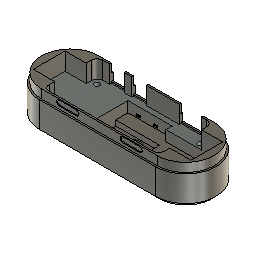
OP_Lower (Autodesk Fusion 360 design; units mm, degrees)
Autodesk Fusion 360 part; units mm, degrees
sketch "Sketch1" plane through (0, 0, 0) normal (0, 0, 1) x (1, 0, 0)
  line L0 (32.75, -17.25) -> (-32.75, -17.25)
  line L1 (-32.75, 17.25) -> (32.75, 17.25)
  arc A0 (-32.75, 17.25) -> (-32.75, -17.25) centre (-32.75, 0) ccw
  arc A1 (32.75, -17.25) -> (32.75, 17.25) centre (32.75, 0) ccw
extrude "Extrude1" add sketch "Sketch1" along normal blind 18
sketch "Sketch2" plane through (0, 0, 18) normal (0, 0, 1) x (-1, 0, 0)
  arc A0 (32.75, -17.25) -> (32.75, 17.25) centre (32.75, 0) ccw
  line L0 (32.75, 17.25) -> (-32.75, 17.25)
  arc A1 (-32.75, 17.25) -> (-32.75, -17.25) centre (-32.75, 0) ccw
  line L1 (-32.75, -17.25) -> (32.75, -17.25)
  line L2 (-12.5, -12.5) -> (12.5, -12.5)
  line L3 (12.5, -12.5) -> (12.5, 12.5)
  line L4 (12.5, 12.5) -> (-12.5, 12.5)
  line L5 (-12.5, 12.5) -> (-12.5, -12.5)
  line L6 (-12.5, -12.5) -> (12.5, 12.5) construction
  line L7 (12.5, -12.5) -> (-12.5, 12.5) construction
  dimension "d9" = 25
  dimension "d10" = 25
  constraint horizontal L2
  constraint perpendicular L2 L3
  constraint parallel L2 L4
  constraint parallel L3 L5
  constraint coincident L6 origin
  constraint coincident L7 origin
  measures "d9" distance of L3.end L4.end
  measures "d10" distance of L2.end L3.end
extrude "Extrude2" cut sketch "Sketch2" against normal blind 15 contours L2 L3 L4 L5
sketch "Sketch3" plane through (0, 0, 3) normal (0, 0, 1) x (-1, 0, 0)
  line L0 (-12.5, 12.5) -> (-12.5, -12.5)
  line L1 (-12.5, -12.5) -> (12.5, -12.5)
  line L2 (12.5, -12.5) -> (12.5, 12.5)
  line L3 (12.5, 12.5) -> (-12.5, 12.5)
sketch "Sketch4" plane through (0, 0, 3) normal (0, 0, 1) x (-1, 0, 0)
  line L0 (-12.5, 12.5) -> (-12.5, -12.5)
  line L1 (-12.5, -12.5) -> (12.5, -12.5)
  line L2 (12.5, -12.5) -> (12.5, 12.5)
  line L3 (12.5, 12.5) -> (-12.5, 12.5)
  line L4 (12.5, 0) -> (12.5, -5.5) construction
  line L5 (12.5, -5.5) -> (-12.5, -5.5)
  line L6 (12.5, 0) -> (12.5, 5.5) construction
  line L7 (12.5, 5.5) -> (-12.5, 5.5)
  constraint midpoint L2 L4.start
  constraint parallel L2 L4
  constraint coincident L0 L5.end
  constraint perpendicular L0 L5
  constraint perpendicular L5 L6
  constraint coincident L0 L7.end
  constraint perpendicular L0 L7
extrude "Extrude4" add sketch "Sketch4" along normal blind 3 contours L0 L2 L3 L7 | L0 L1 L2 L5
sketch "Sketch5" plane through (0, 0, 18) normal (0, 0, 1) x (-1, 0, 0)
  line L0 (12.5, -12.5) -> (-12.5, -12.5)
  line L1 (-12.5, -12.5) -> (-12.5, 12.5)
  line L2 (-12.5, 12.5) -> (12.5, 12.5)
  line L3 (12.5, 12.5) -> (12.5, -12.5)
  arc A0 (32.75, -17.25) -> (32.75, 17.25) centre (32.75, 0) ccw
  line L4 (32.75, 17.25) -> (-32.75, 17.25)
  arc A1 (-32.75, 17.25) -> (-32.75, -17.25) centre (-32.75, 0) ccw
  line L5 (-32.75, -17.25) -> (32.75, -17.25)
  line L6 (29.5, -15.25) -> (25.75, -15.25)
  arc A2 (29.5, -15.25) -> (32.75, -12) centre (29.5, -12) ccw
  line L7 (32.75, 12) -> (32.75, -12)
  arc A3 (32.75, 12) -> (29.5, 15.25) centre (29.5, 12) ccw
  line L8 (-29.5, 15.25) -> (29.5, 15.25)
  arc A4 (-29.5, 15.25) -> (-32.75, 12) centre (-29.5, 12) ccw
  line L9 (-32.75, -12) -> (-32.75, 12)
  arc A5 (-32.75, -12) -> (-29.5, -15.25) centre (-29.5, -12) ccw
  line L10 (-26.35, -15.25) -> (-29.5, -15.25)
  line L11 (-13.85, -17.25) -> (-26.35, -17.25)
  line L12 (-26.35, -17.25) -> (-26.35, -15.25)
  line L13 (-13.85, -15.25) -> (-13.85, -17.25)
  line L14 (4.65, -15.25) -> (-13.85, -15.25)
  line L15 (4.65, -18.25) -> (4.65, -15.25)
  line L16 (13.15, -18.25) -> (4.65, -18.25)
  line L17 (13.15, -15.25) -> (13.15, -18.25)
  line L18 (17.25, -15.25) -> (13.15, -15.25)
  line L19 (17.25, -18.25) -> (17.25, -15.25)
  line L20 (25.75, -18.25) -> (17.25, -18.25)
  line L21 (25.75, -15.25) -> (25.75, -18.25)
  line L22 (32.75, 0) -> (32.75, -9) construction
  line L23 (32.75, 0) -> (32.75, 9) construction
  line L24 (32.75, -9) -> (44.75, -9)
  line L25 (32.75, 9) -> (44.75, 9)
  line L26 (44.75, -9) -> (44.75, 9)
  line L27 (-32.75, 0) -> (-32.75, -9) construction
  line L28 (-32.75, 0) -> (-32.75, 9) construction
  line L29 (-32.75, -9) -> (-44.75, -9)
  line L30 (-32.75, 9) -> (-44.75, 9)
  line L31 (-44.75, 9) -> (-44.75, -9)
  dimension "d20" = 9
  dimension "d21" = 9
  dimension "d23" = 12
  dimension "d26" = 12
  constraint coincident A0.centre L22.start
  constraint parallel L7 L22
  constraint parallel L7 L23
  constraint perpendicular L22 L24
  constraint perpendicular L7 L25
  constraint perpendicular L25 L26
  constraint coincident A1.centre L27.start
  constraint perpendicular L25 L27
  constraint parallel L9 L28
  constraint perpendicular L9 L29
  constraint perpendicular L9 L30
  constraint perpendicular L29 L31
  measures "d20" distance of A0.centre L22.end
  measures "d21" distance of A0.centre L23.end
  measures "d23" distance of L23.end L25.end
  measures "d26" distance of L27.end L29.end
extrude "Extrude5" cut sketch "Sketch5" against normal blind 5 contours L5 L6 A2 L7 A3 L8 A4 L9 A5 L10 L11 L12 L13 L14 L15 L17 L18 L19 L21 | L7 L24 L25 L26 | L9 L29 L30 L31
sketch "Sketch6" plane through (0, 0, 6) normal (0, 0, 1) x (-1, 0, 0)
  line L0 (12.5, 12.5) -> (-12.5, 12.5)
  line L1 (-12.5, 12.5) -> (-12.5, 5.5)
  line L2 (-12.5, 5.5) -> (12.5, 5.5)
  line L3 (12.5, 5.5) -> (12.5, 12.5)
  line L4 (12.5, 5.5) -> (6.5, 5.5) construction
  line L5 (6.5, 5.5) -> (6.5, 12.5)
  dimension "d30" = 6
  constraint coincident L2.end L3.start
  constraint perpendicular L3 L4
  constraint coincident L0 L5.end
  constraint perpendicular L0 L5
  measures "d30" distance of L2.end L4.end
extrude "Extrude6" cut sketch "Sketch6" against normal blind 1.5 contours L0 L2 L3 L5
sketch "Sketch7" plane through (0, 0, 13) normal (0, 0, 1) x (-1, 0, 0)
  line L0 (-12.5, 12.5) -> (12.5, 12.5)
  line L1 (12.5, 12.5) -> (12.5, -12.5)
  line L2 (12.5, -12.5) -> (-12.5, -12.5)
  line L3 (-12.5, -12.5) -> (-12.5, 12.5)
  line L4 (-32.75, 9) -> (-44.75, 9)
  line L5 (-44.75, 9) -> (-44.75, -9)
  line L6 (-44.75, -9) -> (-32.75, -9)
  line L7 (-32.75, -9) -> (-32.75, -12)
  arc A0 (-32.75, -12) -> (-29.5, -15.25) centre (-29.5, -12) ccw
  line L8 (-29.5, -15.25) -> (-26.35, -15.25)
  line L9 (-26.35, -15.25) -> (-26.35, -17.25)
  line L10 (-26.35, -17.25) -> (-13.85, -17.25)
  line L11 (-13.85, -17.25) -> (-13.85, -15.25)
  line L12 (-13.85, -15.25) -> (4.65, -15.25)
  line L13 (4.65, -15.25) -> (4.65, -17.25)
  line L14 (4.65, -17.25) -> (13.15, -17.25)
  line L15 (13.15, -17.25) -> (13.15, -15.25)
  line L16 (13.15, -15.25) -> (17.25, -15.25)
  line L17 (17.25, -15.25) -> (17.25, -17.25)
  line L18 (17.25, -17.25) -> (25.75, -17.25)
  line L19 (25.75, -17.25) -> (25.75, -15.25)
  line L20 (25.75, -15.25) -> (29.5, -15.25)
  arc A1 (29.5, -15.25) -> (32.75, -12) centre (29.5, -12) ccw
  line L21 (32.75, -12) -> (32.75, -9)
  line L22 (32.75, -9) -> (44.75, -9)
  line L23 (44.75, -9) -> (44.75, 9)
  line L24 (44.75, 9) -> (32.75, 9)
  line L25 (32.75, 9) -> (32.75, 12)
  arc A2 (32.75, 12) -> (29.5, 15.25) centre (29.5, 12) ccw
  line L26 (29.5, 15.25) -> (-29.5, 15.25)
  arc A3 (-29.5, 15.25) -> (-32.75, 12) centre (-29.5, 12) ccw
  line L27 (-32.75, 12) -> (-32.75, 9)
  line L28 (0, 15.25) -> (26.5, 15.25) construction
  line L29 (0, 15.25) -> (-26.5, 15.25) construction
  line L30 (26.5, 15.25) -> (26.5, 9.25)
  line L31 (-26.5, 15.25) -> (-26.5, 9.25)
  line L32 (26.5, 9.25) -> (-26.5, 9.25)
  dimension "d33" = 26.5
  dimension "d34" = 26.5
  dimension "d35" = 6
  dimension "d36" = 6
  constraint midpoint L26 L28.start
  constraint parallel L26 L28
  constraint parallel L26 L29
  constraint perpendicular L28 L30
  constraint perpendicular L29 L31
  measures "d33" distance of L28.start L28.end
  measures "d34" distance of L28.start L29.end
  measures "d35" distance of L28.end L30.end
  measures "d36" distance of L29.end L31.end
extrude "Extrude7" cut sketch "Sketch7" against normal blind 4 contours L0 L1 L3 L26 L30 L31 L32
sketch "Sketch8" plane through (0, 0, 13) normal (0, 0, 1) x (-1, 0, 0)
  line L0 (26.5, 9.25) -> (12.5, 9.25)
  line L1 (12.5, 9.25) -> (12.5, -12.5)
  line L2 (12.5, -12.5) -> (-12.5, -12.5)
  line L3 (-12.5, -12.5) -> (-12.5, 9.25)
  line L4 (-12.5, 9.25) -> (-26.5, 9.25)
  line L5 (-26.5, 9.25) -> (-26.5, 15.25)
  line L6 (-26.5, 15.25) -> (-29.5, 15.25)
  arc A0 (-29.5, 15.25) -> (-32.75, 12) centre (-29.5, 12) ccw
  line L7 (-32.75, 12) -> (-32.75, 9)
  line L8 (-32.75, 9) -> (-44.75, 9)
  line L9 (-44.75, 9) -> (-44.75, -9)
  line L10 (-44.75, -9) -> (-32.75, -9)
  line L11 (-32.75, -9) -> (-32.75, -12)
  arc A1 (-32.75, -12) -> (-29.5, -15.25) centre (-29.5, -12) ccw
  line L12 (-29.5, -15.25) -> (-26.35, -15.25)
  line L13 (-26.35, -15.25) -> (-26.35, -17.25)
  line L14 (-26.35, -17.25) -> (-13.85, -17.25)
  line L15 (-13.85, -17.25) -> (-13.85, -15.25)
  line L16 (-13.85, -15.25) -> (4.65, -15.25)
  line L17 (4.65, -15.25) -> (4.65, -17.25)
  line L18 (4.65, -17.25) -> (13.15, -17.25)
  line L19 (13.15, -17.25) -> (13.15, -15.25)
  line L20 (13.15, -15.25) -> (17.25, -15.25)
  line L21 (17.25, -15.25) -> (17.25, -17.25)
  line L22 (17.25, -17.25) -> (25.75, -17.25)
  line L23 (25.75, -17.25) -> (25.75, -15.25)
  line L24 (25.75, -15.25) -> (29.5, -15.25)
  arc A2 (29.5, -15.25) -> (32.75, -12) centre (29.5, -12) ccw
  line L25 (32.75, -12) -> (32.75, -9)
  line L26 (32.75, -9) -> (44.75, -9)
  line L27 (44.75, -9) -> (44.75, 9)
  line L28 (44.75, 9) -> (32.75, 9)
  line L29 (32.75, 9) -> (32.75, 12)
  arc A3 (32.75, 12) -> (29.5, 15.25) centre (29.5, 12) ccw
  line L30 (29.5, 15.25) -> (26.5, 15.25)
  line L31 (26.5, 15.25) -> (26.5, 9.25)
  line L32 (-32.75, -9) -> (-12.5, -9)
  line L33 (-32.75, 9) -> (-12.5, 9)
  constraint horizontal L32
  constraint coincident L10.end L11.start
  constraint coincident L3 L32.end
  constraint horizontal L33
  constraint coincident L7.end L8.start
  constraint coincident L3 L33.end
extrude "Extrude8" cut sketch "Sketch8" against normal up to surface (7 mm away) contours L3 L8 L9 L10 L32 L33
sketch "Sketch9" plane through (0, 0, 13) normal (0, 0, 1) x (-1, 0, 0)
  line L0 (-32.75, 9) -> (-12.5, 9)
  line L1 (-12.5, 9) -> (-12.5, 9.25)
  line L2 (-12.5, 9.25) -> (-26.5, 9.25)
  line L3 (-26.5, 9.25) -> (-26.5, 15.25)
  line L4 (-26.5, 15.25) -> (-29.5, 15.25)
  arc A0 (-29.5, 15.25) -> (-32.75, 12) centre (-29.5, 12) ccw
  line L5 (-32.75, 12) -> (-32.75, 9)
  line L6 (-26.5, 9.25) -> (-26.5, 9)
  constraint vertical L6
  constraint coincident L2.end L3.start
  constraint coincident L0 L6.end
extrude "Extrude9" cut sketch "Sketch9" against normal up to surface (7 mm away) contours L0 L1 L2 L6
sketch "Sketch10" plane through (0, 12.5, 0) normal (0, -1, 0) x (1, 0, 0)
  line L0 (12.5, 13) -> (-12.5, 13)
  line L1 (-12.5, 13) -> (-12.5, 6)
  line L2 (-12.5, 6) -> (12.5, 6)
  line L3 (12.5, 6) -> (12.5, 13)
  line L4 (-12.5, 6) -> (-7.5, 6) construction
  line L5 (-7.5, 6) -> (-7.5, 7) construction
  line L6 (-7.5, 7) -> (-5.5, 7)
  line L7 (-5.5, 7) -> (-5.5, 8)
  line L8 (-5.5, 8) -> (-7.5, 8)
  line L9 (-7.5, 8) -> (-7.5, 7)
  line L10 (-5.5, 7) -> (2.5, 7) construction
  line L11 (2.5, 7) -> (4.5, 7)
  line L12 (4.5, 7) -> (4.5, 8)
  line L13 (4.5, 8) -> (2.5, 8)
  line L14 (2.5, 8) -> (2.5, 7)
  dimension "d44" = 1
  dimension "d45" = 2
  dimension "d46" = 1
  dimension "d47" = 8
  dimension "d48" = 2
  dimension "d49" = 1
  constraint coincident L1.end L2.start
  constraint perpendicular L1 L4
  constraint perpendicular L4 L5
  constraint horizontal L6
  constraint vertical L7
  constraint horizontal L8
  constraint vertical L9
  constraint perpendicular L7 L10
  constraint horizontal L11
  constraint vertical L12
  constraint horizontal L13
  constraint vertical L14
  measures "d44" distance of L4.end L5.end
  measures "d45" distance of L5.end L6.end
  measures "d46" distance of L5.end L8.end
  measures "d47" distance of L6.end L10.end
  measures "d48" distance of L10.end L11.end
  measures "d49" distance of L10.end L13.end
extrude "Extrude10" add sketch "Sketch10" along normal blind 0.5 contours L6 L7 L8 L9 | L11 L12 L13 L14
chamfer "Chamfer1" distance 0.2 distance2 0.2 4 edges at (-6.5, 12, 8) (-6.5, 12, 7) (3.5, 12, 8) (3.5, 12, 7) measured on face at (-6.8333, 12, 7.6667) measured on face at (-6.8333, 12, 7.6667) measured on face at (3.1667, 12, 7.6667) measured on face at (3.1667, 12, 7.6667)
sketch "Sketch11" plane through (0, -12.5, 0) normal (0, 1, 0) x (-1, 0, 0)
  line L0 (12.5, 9) -> (-12.5, 9)
  line L1 (-12.5, 9) -> (-12.5, 6)
  line L2 (-12.5, 6) -> (6.5, 6)
  line L3 (6.5, 6) -> (6.5, 4.5)
  line L4 (6.5, 4.5) -> (12.5, 4.5)
  line L5 (12.5, 4.5) -> (12.5, 9)
  line L6 (6.5, 6) -> (12.5, 6) construction
  line L7 (12.5, 6) -> (12.5, 7) construction
  line L8 (12.5, 7) -> (7.5, 7) construction
  line L9 (7.5, 7) -> (5.5, 7)
  line L10 (5.5, 7) -> (5.5, 8)
  line L11 (5.5, 8) -> (7.5, 8)
  line L12 (7.5, 8) -> (7.5, 7)
  line L13 (5.5, 7) -> (-2.5, 7) construction
  line L14 (-2.5, 7) -> (-4.5, 7)
  line L15 (-4.5, 7) -> (-4.5, 8)
  line L16 (-4.5, 8) -> (-2.5, 8)
  line L17 (-2.5, 8) -> (-2.5, 7)
  dimension "d54" = 1
  dimension "d55" = 5
  dimension "d56" = 2
  dimension "d57" = 1
  dimension "d58" = 8
  dimension "d59" = 2
  dimension "d60" = 1
  constraint coincident L2.end L3.start
  constraint coincident L5 L6.end
  constraint perpendicular L5 L6
  constraint perpendicular L6 L7
  constraint perpendicular L7 L8
  constraint horizontal L9
  constraint vertical L10
  constraint horizontal L11
  constraint vertical L12
  constraint perpendicular L10 L13
  constraint horizontal L14
  constraint vertical L15
  constraint horizontal L16
  constraint vertical L17
  measures "d54" distance of L6.end L7.end
  measures "d55" distance of L7.end L8.end
  measures "d56" distance of L8.end L9.end
  measures "d57" distance of L8.end L11.end
  measures "d58" distance of L9.end L13.end
  measures "d59" distance of L13.end L14.end
  measures "d60" distance of L13.end L16.end
extrude "Extrude11" add sketch "Sketch11" along normal blind 0.5 contours L9 L10 L11 L12 | L14 L15 L16 L17
chamfer "Chamfer2" distance 0.2 distance2 0.2 4 edges at (-6.5, -12, 8) (-6.5, -12, 7) (3.5, -12, 8) (3.5, -12, 7) measured on face at (-6.1667, -12, 7.6667) measured on face at (-6.1667, -12, 7.6667) measured on face at (3.8333, -12, 7.6667) measured on face at (3.8333, -12, 7.6667)
sketch "Sketch13" plane through (0, 0, 18) normal (0, 0, 1) x (-1, 0, 0)
  line L0 (-26.35, -17.25) -> (-26.35, -15.25)
  line L1 (-26.35, -15.25) -> (-29.5, -15.25)
  arc A0 (-32.75, -12) -> (-29.5, -15.25) centre (-29.5, -12) ccw
  line L2 (-32.75, -12) -> (-32.75, -9)
  line L3 (-32.75, -9) -> (-44.75, -9)
  line L4 (-44.75, -9) -> (-44.75, 9)
  line L5 (-44.75, 9) -> (-32.75, 9)
  line L6 (-32.75, 9) -> (-32.75, 12)
  arc A1 (-29.5, 15.25) -> (-32.75, 12) centre (-29.5, 12) ccw
  line L7 (-29.5, 15.25) -> (29.5, 15.25)
  arc A2 (32.75, 12) -> (29.5, 15.25) centre (29.5, 12) ccw
  line L8 (32.75, 12) -> (32.75, 9)
  line L9 (32.75, 9) -> (44.75, 9)
  line L10 (44.75, 9) -> (44.75, -9)
  line L11 (44.75, -9) -> (32.75, -9)
  line L12 (32.75, -9) -> (32.75, -12)
  arc A3 (29.5, -15.25) -> (32.75, -12) centre (29.5, -12) ccw
  line L13 (29.5, -15.25) -> (25.75, -15.25)
  line L14 (25.75, -15.25) -> (25.75, -17.25)
  line L15 (25.75, -17.25) -> (32.75, -17.25)
  arc A4 (32.75, -17.25) -> (32.75, 17.25) centre (32.75, 0) ccw
  line L16 (32.75, 17.25) -> (-32.75, 17.25)
  arc A5 (-32.75, 17.25) -> (-32.75, -17.25) centre (-32.75, 0) ccw
  line L17 (-32.75, -17.25) -> (-26.35, -17.25)
  line L18 (25.75, -16.25) -> (32.75, -16.25)
  arc A6 (32.75, -16.25) -> (32.75, 16.25) centre (32.75, 0) ccw
  line L19 (32.75, 16.25) -> (-32.75, 16.25)
  arc A7 (-32.75, 16.25) -> (-32.75, -16.25) centre (-32.75, 0) ccw
  line L20 (-32.75, -16.25) -> (-26.35, -16.25)
  line L21 (25.75, -15.25) -> (32.75, -15.25)
  arc A8 (32.75, -15.25) -> (32.75, 15.25) centre (32.75, 0) ccw
  line L22 (32.75, 15.25) -> (-32.75, 15.25)
  arc A9 (-32.75, 15.25) -> (-32.75, -15.25) centre (-32.75, 0) ccw
  line L23 (-32.75, -15.25) -> (-26.35, -15.25)
  dimension "d79" = -1
  dimension "d80" = -2
extrude "Extrude13" add sketch "Sketch13" along normal blind 2 contours L0 L1 L7 L13 L14 L18 A6 L19 A7 L20 L21 A8 L22 A9 L23
sketch "Sketch14" plane through (0, 0, 18) normal (0, 0, 1) x (-1, 0, 0)
  line L0 (-13.85, -15.25) -> (-13.85, -17.25)
  line L1 (-13.85, -17.25) -> (4.65, -17.25)
  line L2 (4.65, -17.25) -> (4.65, -15.25)
  line L3 (4.65, -15.25) -> (-13.85, -15.25)
  line L4 (4.65, -16.25) -> (-13.85, -16.25)
  constraint midpoint L2 L4.start
  constraint midpoint L0 L4.end
extrude "Extrude14" add sketch "Sketch14" along normal blind 2 contours L0 L2 L3 L4
sketch "Sketch15" plane through (0, 0, 18) normal (0, 0, 1) x (-1, 0, 0)
  line L0 (13.15, -15.25) -> (13.15, -17.25)
  line L1 (13.15, -17.25) -> (17.25, -17.25)
  line L2 (17.25, -17.25) -> (17.25, -15.25)
  line L3 (17.25, -15.25) -> (13.15, -15.25)
  line L4 (17.25, -16.25) -> (13.15, -16.25)
  constraint midpoint L2 L4.start
  constraint midpoint L0 L4.end
extrude "Extrude15" add sketch "Sketch15" along normal blind 2 contours L0 L2 L3 L4
sketch "Sketch16" plane through (0, 0, 0) normal (0, 0, -1) x (1, 0, 0)
  circle A0 centre (-29.25, 11.75) radius 2.5
  circle A1 centre (-29.25, -11.75) radius 2.5
  circle A2 centre (29.25, 11.75) radius 2.5
  circle A3 centre (29.25, -11.75) radius 2.5
  arc A4 (-32.75, 17.25) -> (-32.75, -17.25) centre (-32.75, 0) ccw
  line L0 (-32.75, -17.25) -> (32.75, -17.25)
  arc A5 (32.75, -17.25) -> (32.75, 17.25) centre (32.75, 0) ccw
  line L1 (32.75, 17.25) -> (-32.75, 17.25)
  dimension "d88" = 5
  dimension "d89" = 5
  dimension "d90" = 5
  dimension "d91" = 5
  measures "d88" diameter of A0
  measures "d89" diameter of A1
  measures "d90" diameter of A2
  measures "d91" diameter of A3
sketch "Sketch17" plane through (0, 0, 13) normal (0, 0, 1) x (-1, 0, 0)
  line L0 (-12.5, -9) -> (-32.75, -9)
  line L1 (-32.75, -9) -> (-32.75, -12)
  arc A0 (-32.75, -12) -> (-29.5, -15.25) centre (-29.5, -12) ccw
  line L2 (-29.5, -15.25) -> (-26.35, -15.25)
  line L3 (-26.35, -15.25) -> (-26.35, -17.25)
  line L4 (-26.35, -17.25) -> (-13.85, -17.25)
  line L5 (-13.85, -17.25) -> (-13.85, -15.25)
  line L6 (-13.85, -15.25) -> (4.65, -15.25)
  line L7 (4.65, -15.25) -> (4.65, -17.25)
  line L8 (4.65, -17.25) -> (13.15, -17.25)
  line L9 (13.15, -17.25) -> (13.15, -15.25)
  line L10 (13.15, -15.25) -> (17.25, -15.25)
  line L11 (17.25, -15.25) -> (17.25, -17.25)
  line L12 (17.25, -17.25) -> (25.75, -17.25)
  line L13 (25.75, -17.25) -> (25.75, -15.25)
  line L14 (25.75, -15.25) -> (29.5, -15.25)
  arc A1 (29.5, -15.25) -> (32.75, -12) centre (29.5, -12) ccw
  line L15 (32.75, -12) -> (32.75, -9)
  line L16 (32.75, -9) -> (44.75, -9)
  line L17 (44.75, -9) -> (44.75, 9)
  line L18 (44.75, 9) -> (32.75, 9)
  line L19 (32.75, 9) -> (32.75, 12)
  arc A2 (32.75, 12) -> (29.5, 15.25) centre (29.5, 12) ccw
  line L20 (29.5, 15.25) -> (26.5, 15.25)
  line L21 (26.5, 15.25) -> (26.5, 9.25)
  line L22 (26.5, 9.25) -> (12.5, 9.25)
  line L23 (12.5, 9.25) -> (12.5, -12.5)
  line L24 (12.5, -12.5) -> (-12.5, -12.5)
  line L25 (-12.5, -12.5) -> (-12.5, -9)
  line L26 (25.75, -16.25) -> (17.25, -16.25)
  line L27 (13.15, -16.25) -> (4.65, -16.25)
  line L28 (-13.85, -16.25) -> (-26.35, -16.25)
  point P0 (25.75, -16.25)
  point P1 (17.25, -16.25)
  point P2 (13.15, -16.25)
  point P3 (4.65, -16.25)
  point P4 (-13.85, -16.25)
  point P5 (-26.35, -16.25)
  constraint coincident P0 L26.start
  constraint coincident P1 L26.end
  constraint coincident P2 L27.start
  constraint coincident P3 L27.end
  constraint coincident P4 L28.start
  constraint coincident P5 L28.end
extrude "Extrude17" add sketch "Sketch17" along normal blind 0.8 contours L7 L8 L9 L27 | L11 L12 L13 L26
sketch "Sketch18" plane through (0, 0, 13) normal (0, 0, 1) x (-1, 0, 0)
  line L0 (4.65, -16.25) -> (13.15, -16.25)
  line L1 (13.15, -16.25) -> (13.15, -15.25)
  line L2 (13.15, -15.25) -> (17.25, -15.25)
  line L3 (17.25, -15.25) -> (17.25, -16.25)
  line L4 (17.25, -16.25) -> (25.75, -16.25)
  line L5 (25.75, -16.25) -> (25.75, -15.25)
  line L6 (25.75, -15.25) -> (29.5, -15.25)
  arc A0 (29.5, -15.25) -> (32.75, -12) centre (29.5, -12) ccw
  line L7 (32.75, -12) -> (32.75, -9)
  line L8 (32.75, -9) -> (44.75, -9)
  line L9 (44.75, -9) -> (44.75, 9)
  line L10 (44.75, 9) -> (32.75, 9)
  line L11 (32.75, 9) -> (32.75, 12)
  arc A1 (32.75, 12) -> (29.5, 15.25) centre (29.5, 12) ccw
  line L12 (29.5, 15.25) -> (26.5, 15.25)
  line L13 (26.5, 15.25) -> (26.5, 9.25)
  line L14 (26.5, 9.25) -> (12.5, 9.25)
  line L15 (12.5, 9.25) -> (12.5, -12.5)
  line L16 (12.5, -12.5) -> (-12.5, -12.5)
  line L17 (-12.5, -12.5) -> (-12.5, -9)
  line L18 (-12.5, -9) -> (-32.75, -9)
  line L19 (-32.75, -9) -> (-32.75, -12)
  arc A2 (-32.75, -12) -> (-29.5, -15.25) centre (-29.5, -12) ccw
  line L20 (-29.5, -15.25) -> (-26.35, -15.25)
  line L21 (-26.35, -15.25) -> (-26.35, -17.25)
  line L22 (-26.35, -17.25) -> (-13.85, -17.25)
  line L23 (-13.85, -17.25) -> (-13.85, -15.25)
  line L24 (-13.85, -15.25) -> (4.65, -15.25)
  line L25 (4.65, -15.25) -> (4.65, -16.25)
  line L26 (-13.85, -16.25) -> (-26.35, -16.25)
  point P0 (-13.85, -16.25)
  point P1 (-26.35, -16.25)
  constraint coincident P0 L26.start
  constraint coincident P1 L26.end
extrude "Extrude18" add sketch "Sketch18" along normal up to surface (5 mm away) contours L21 L22 L23 L26
sketch "Sketch19" plane through (0, 0, 3) normal (0, 0, 1) x (-1, 0, 0)
  line L0 (12.5, 5.5) -> (-12.5, 5.5)
  line L1 (-12.5, 5.5) -> (-12.5, -5.5)
  line L2 (-12.5, -5.5) -> (12.5, -5.5)
  line L3 (12.5, -5.5) -> (12.5, 5.5)
  circle A0 centre (-2, 0) radius 4.75
  dimension "d99" = 9.5
  measures "d99" diameter of A0
extrude "Extrude19" cut sketch "Sketch19" against normal up to surface (3 mm away) contours A0
chamfer "Chamfer5" distance 1 angle 45 1 edges at (6.4286, 1.7177, 0)
extrude "Extrude20" add 3 faces at (10.9167, -15.5833, 20) (1.5167, 15.9167, 20) (-15.8833, 15.9167, 20) along direction (0, 0, 1) blind 2
sketch "Sketch20" plane through (0, 16.25, 0) normal (0, 1, 0) x (-1, 0, 0)
  line L0 (-13.85, 18) -> (4.65, 18)
  line L1 (4.65, 18) -> (4.65, 22)
  line L2 (4.65, 22) -> (-13.85, 22)
  line L3 (-13.85, 22) -> (-13.85, 18)
  line L4 (-13.85, 20) -> (-10.85, 20) construction
  line L5 (4.65, 20) -> (1.65, 20) construction
  line L6 (1.65, 20) -> (0.15, 20) construction
  line L7 (0.15, 20) -> (0.15, 21.5) construction
  line L8 (0.15, 20) -> (0.15, 18.5) construction
  arc A0 (0.15, 18.5) -> (0.15, 21.5) centre (0.15, 20) ccw
  line L9 (-10.85, 20) -> (-9.35, 20) construction
  line L10 (-9.35, 20) -> (-9.35, 21.5) construction
  line L11 (-9.35, 20) -> (-9.35, 18.5) construction
  arc A1 (-9.35, 21.5) -> (-9.35, 18.5) centre (-9.35, 20) ccw
  line L12 (0.15, 21.5) -> (-9.35, 21.5)
  line L13 (0.15, 18.5) -> (-9.35, 18.5)
  dimension "d105" = 3
  dimension "d106" = 3
  dimension "d110" = 1.5
  dimension "d111" = 1.5
  dimension "d112" = 1.5
  dimension "d113" = 1.5
  dimension "d114" = 1.5
  dimension "d115" = 1.5
  constraint midpoint L3 L4.start
  constraint perpendicular L3 L4
  constraint midpoint L1 L5.start
  constraint perpendicular L1 L5
  constraint parallel L5 L6
  constraint perpendicular L6 L7
  constraint perpendicular L6 L8
  constraint coincident L5.end A0
  constraint parallel L4 L9
  constraint perpendicular L9 L10
  constraint perpendicular L9 L11
  constraint coincident L4.end A1
  measures "d105" distance of L4.start L4.end
  measures "d106" distance of L5.start L5.end
  measures "d110" distance of L5.end L6.end
  measures "d111" distance of L6.end L7.end
  measures "d112" distance of L6.end L8.end
  measures "d113" distance of L4.end L9.end
  measures "d114" distance of L9.end L10.end
  measures "d115" distance of L9.end L11.end
extrude "Extrude21" cut sketch "Sketch20" against normal blind 0.3 contours A0 A1 L12 L13
chamfer "Chamfer8" distance 0.3 angle 45 4 edges at (4.6, 15.95, 18.5) (10.85, 15.95, 20) (4.6, 15.95, 21.5) (-1.65, 15.95, 20)
sketch "Sketch21" plane through (0, -16.25, 0) normal (0, -1, 0) x (1, 0, 0)
  line L0 (-32.75, 18) -> (32.75, 18)
  line L1 (32.75, 18) -> (32.75, 22)
  line L2 (32.75, 22) -> (-32.75, 22)
  line L3 (-32.75, 22) -> (-32.75, 18)
  line L4 (13.25, 21.5) -> (22.75, 21.5)
  arc A0 (13.25, 21.5) -> (13.25, 18.5) centre (13.25, 20) ccw
  line L5 (22.75, 18.5) -> (13.25, 18.5)
  arc A1 (22.75, 18.5) -> (22.75, 21.5) centre (22.75, 20) ccw
  line L6 (-32.75, 20) -> (-22.75, 20) construction
  line L7 (32.75, 20) -> (22.75, 20) construction
  line L8 (-22.75, 21.5) -> (-13.25, 21.5)
  arc A2 (-22.75, 21.5) -> (-22.75, 18.5) centre (-22.75, 20) ccw
  line L9 (-13.25, 18.5) -> (-22.75, 18.5)
  arc A3 (-13.25, 18.5) -> (-13.25, 21.5) centre (-13.25, 20) ccw
  dimension "d119" = 10
  dimension "d120" = 10
  constraint midpoint L3 L6.start
  constraint perpendicular L3 L6
  constraint midpoint L1 L7.start
  constraint perpendicular L1 L7
  measures "d119" distance of L6.start L6.end
  measures "d120" distance of L7.start A1.centre
extrude "Extrude22" cut sketch "Sketch21" against normal blind 0.3 contours L4 A0 L5 A1 | L8 A2 L9 A3
chamfer "Chamfer7" distance 0.3 angle 45 8 edges at (11.75, -15.95, 20) (18, -15.95, 21.5) (24.25, -15.95, 20) (18, -15.95, 18.5) (-18, -15.95, 18.5) (-24.25, -15.95, 20) (-18, -15.95, 21.5) (-11.75, -15.95, 20)
extrude "Extrude24" add 2 faces at (-45.4819, 1.8572, 18) (45.4819, -1.8572, 18) along direction (0, 0, 1) blind 4
chamfer "Chamfer9" distance 2.4 angle 45 4 edges at (0, 17.25, 0) (50, 0, 0) (0, -17.25, 0) (-50, 0, 0) measured on face at (-23.0833, 0, 0) measured on face at (48.4735, 7.0947, 6) measured on face at (-23.0833, 0, 0) measured on face at (-45.6837, -11.4141, 6)
sketch "Sketch24" plane through (0, 0, 18) normal (0, 0, 1) x (-1, 0, 0)
  line L0 (-26.35, -16.25) -> (-32.75, -16.25)
  arc A0 (-32.75, 16.25) -> (-32.75, -16.25) centre (-32.75, 0) ccw
  line L1 (-32.75, 16.25) -> (32.75, 16.25)
  arc A1 (32.75, -16.25) -> (32.75, 16.25) centre (32.75, 0) ccw
  line L2 (32.75, -16.25) -> (25.75, -16.25)
  line L3 (25.75, -16.25) -> (25.75, -17.25)
  line L4 (25.75, -17.25) -> (32.75, -17.25)
  arc A2 (32.75, -17.25) -> (32.75, 17.25) centre (32.75, 0) ccw
  line L5 (32.75, 17.25) -> (-32.75, 17.25)
  arc A3 (-32.75, 17.25) -> (-32.75, -17.25) centre (-32.75, 0) ccw
  line L6 (-32.75, -17.25) -> (4.65, -17.25)
  line L7 (4.65, -17.25) -> (4.65, -16.25)
  line L8 (4.65, -16.25) -> (-13.85, -16.25)
  line L9 (-13.85, -16.25) -> (-26.35, -16.25)
  line L10 (-13.85, -16.25) -> (-13.85, -17.25)
  line L11 (-26.35, -16.25) -> (-26.35, -17.25)
  constraint vertical L10
  constraint coincident L8.end L9.start
  constraint coincident L6 L10.end
  constraint coincident L0.start L9.end
  constraint coincident L6 L11.end
extrude "Extrude27" cut 2 faces at (29.5833, -12.0833, 13) (-23.9167, 4.0833, 13) along direction (0, 0, -1) blind 1
sketch "Sketch25" plane through (0, 0, 0) normal (0, 0, -1) x (1, 0, 0)
  circle A0 centre (2, 0) radius 5.75
  line L0 (-32.75, -14.85) -> (32.75, -14.85)
  arc A1 (32.75, -14.85) -> (32.75, 14.85) centre (32.75, 0) ccw
  line L1 (32.75, 14.85) -> (-32.75, 14.85)
  arc A2 (-32.75, 14.85) -> (-32.75, -14.85) centre (-32.75, 0) ccw
  circle A3 centre (-29.25, -11.75) radius 2.5
  circle A4 centre (-29.25, 11.75) radius 2.5
  circle A5 centre (29.25, 11.75) radius 2.5
  circle A6 centre (29.25, -11.75) radius 2.5
  circle A7 centre (-29.25, 11.75) radius 1.5
  circle A8 centre (-29.25, -11.75) radius 1.5
  circle A9 centre (29.25, 11.75) radius 1.5
  circle A10 centre (29.25, -11.75) radius 1.5
  dimension "d216" = 3
  dimension "d217" = 3
  dimension "d218" = 3
  dimension "d219" = 3
  constraint concentric A4 A7
  constraint concentric A3 A8
  constraint concentric A5 A9
  constraint concentric A6 A10
  measures "d216" diameter of A7
  measures "d217" diameter of A8
  measures "d218" diameter of A9
  measures "d219" diameter of A10
extrude "Extrude28" cut sketch "Sketch25" against normal up to surface (12 mm away) contours A7 | A8 | A9 | A10
extrude "Extrude29" cut sketch "Sketch25" against normal blind 7 contours A3 | A4 | A5 | A6
chamfer "Chamfer10" distance 1 angle 45 4 edges at (-31.5808, -12.654, 7) (-31.5808, 10.846, 7) (26.9192, -12.654, 7) (26.9192, 10.846, 7)
extrude "Extrude30" cut 2 faces at (-7.4833, 16.9167, 13.8) (-20.0833, 16.5833, 13.8) along direction (0, 0, -1) blind 1
extrude "Extrude31" cut sketch "Sketch24" against normal up to surface (5.2 mm away) contours L6 L9 L10 L11
sketch "Sketch26" plane through (0, 0, 12) normal (0, 0, 1) x (-1, 0, 0)
  circle A0 centre (29.25, -11.75) radius 1.5
  circle A1 centre (-29.25, -11.75) radius 1.5
  circle A2 centre (29.25, 11.75) radius 1.5
  line L0 (-26.35, -16.25) -> (-13.85, -16.25)
  line L1 (-13.85, -16.25) -> (-13.85, -15.25)
  line L2 (-13.85, -15.25) -> (4.65, -15.25)
  line L3 (4.65, -15.25) -> (4.65, -16.25)
  line L4 (4.65, -16.25) -> (13.15, -16.25)
  line L5 (13.15, -16.25) -> (13.15, -15.25)
  line L6 (13.15, -15.25) -> (17.25, -15.25)
  line L7 (17.25, -15.25) -> (17.25, -16.25)
  line L8 (17.25, -16.25) -> (25.75, -16.25)
  line L9 (25.75, -16.25) -> (25.75, -15.25)
  line L10 (25.75, -15.25) -> (29.5, -15.25)
  arc A3 (29.5, -15.25) -> (32.75, -12) centre (29.5, -12) ccw
  line L11 (32.75, -12) -> (32.75, -9)
  line L12 (32.75, -9) -> (44.75, -9)
  line L13 (44.75, -9) -> (44.75, 9)
  line L14 (44.75, 9) -> (32.75, 9)
  line L15 (32.75, 9) -> (32.75, 12)
  arc A4 (32.75, 12) -> (29.5, 15.25) centre (29.5, 12) ccw
  line L16 (29.5, 15.25) -> (26.5, 15.25)
  line L17 (26.5, 15.25) -> (26.5, 9.25)
  line L18 (26.5, 9.25) -> (12.5, 9.25)
  line L19 (12.5, 9.25) -> (12.5, -12.5)
  line L20 (12.5, -12.5) -> (-12.5, -12.5)
  line L21 (-12.5, -12.5) -> (-12.5, -9)
  line L22 (-12.5, -9) -> (-32.75, -9)
  line L23 (-32.75, -9) -> (-32.75, -12)
  arc A5 (-32.75, -12) -> (-29.5, -15.25) centre (-29.5, -12) ccw
  line L24 (-29.5, -15.25) -> (-26.35, -15.25)
  line L25 (-26.35, -15.25) -> (-26.35, -16.25)
extrude "Extrude32" cut 3 faces at (-10.9167, -16.5833, 18) (7.6833, 16.5833, 18) (-14.5167, 16.5833, 18) along direction (0, 0, -1) blind 1
